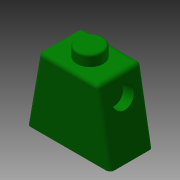
# Autodesk Inventor part: TORSO
Saved by Autodesk Inventor 2015 (Build 190159000, 159)
## iProperties
Created: 2012-05-01
Part Number: TORSO
Material: 250
Document SubType Name: Modeling
Mass: 8.54388 g
Surface Area: 9.94127 cm^2
Volume: 1.08839 cm^3
Density: 7.85 g/cm^3
Appearance: Steel
Autodesk Inventor part; units mm, degrees
ref_plane "YZ Plane" through (0, 0, 0) normal (1, 0, 0) x (0, 1, 0)
ref_plane "XZ Plane" through (0, 0, 0) normal (0, 1, 0) x (-1, 0, 0)
ref_plane "XY Plane" through (0, 0, 0) normal (0, 0, 1) x (1, 0, 0)
sketch "Sketch1" plane through (0, 0, 0) normal (0, 0, 1) x (1, 0, 0)
  line L0 (-7.72, -6.385) -> (7.72, -6.385)
  line L1 (7.72, -6.385) -> (5.4683, 6.385)
  line L2 (5.4683, 6.385) -> (-5.4683, 6.385)
  line L3 (-5.4683, 6.385) -> (-7.72, -6.385)
  point P0 (0, 0)
  point P1 (0, -6.385)
  point P2 (-6.5942, 0)
  dimension "d0" = 15.44
  dimension "d1" = 80
  dimension "d2" = 12.77
  constraints: 8 end point, 2 midpoint, 1 equal length, 1 horizontal, 1 horizontal alignment, 1 parallel, 1 vertical alignment
  measures "d0" distance of L0.start L0.end
  measures "d1" angle of L1 L0
  measures "d2" distance between parallel lines of L2 L0
extrude "Extrusion1" add sketch "Sketch1" along normal mid plane 8
sketch "Sketch2" plane through (-7.72, -6.385, 4) normal (0, -1, 0) x (1, 0, 0)
  line L0 (15.44, -8) -> (15.44, 0) projected
  line L1 (3.72, -4) -> (11.72, -4) construction
  circle A0 centre (3.72, -4) radius 2.5
  circle A1 centre (11.72, -4) radius 2.5
  point P0 (7.72, -4)
  point P1 (7.72, -4)
  dimension "d5" = 5
  dimension "d6" = 8
  constraints: 3 coincident, 2 centre point, 2 end point, 1 equal radius, 1 midpoint, 1 perpendicular
  measures "d5" diameter of A0
  measures "d6" distance of L1.start L1.end
extrude "Extrusion2" cut sketch "Sketch2" against normal blind 6
sketch "Sketch3" plane through (-5.4683, 6.385, 4) normal (0, 1, 0) x (1, 0, 0)
  circle A0 centre (5.4683, 4) radius 2.44
  dimension "d9" = 4.88
  constraints: 1 centre point, 1 coincident
  measures "d9" diameter of A0
extrude "Extrusion3" add sketch "Sketch3" along normal blind 2
fillet "Fillet1" radius 0.4 1 edges at (-2.44, 8.385, 0)
fillet "Fillet2" radius 0.75 4 edges at (-6.5942, 0, 4) (-6.5942, 0, -4) (6.5942, 0, -4) (6.5942, 0, 4)
fillet "Fillet3" radius 0.75 8 edges at (-5.2452, 6.385, -3.7803) (-5.4683, 6.385, 0) (-5.2452, 6.385, 3.7803) (0, 6.385, 4) (5.2452, 6.385, 3.7803) (5.4683, 6.385, 0) (5.2452, 6.385, -3.7803) (0, 6.385, -4)
sketch "Sketch4" plane through (-7.72, -6.385, -3.25) normal (-0.9848, 0.1736, 0) x (0, 0, 1)
  line L0 (6.5, 0) -> (0, 0) projected
  circle A0 centre (3.25, 9.5) radius 2
  point P0 (3.25, 7.6286)
  dimension "d15" = 4
  dimension "d16" = 9.5
  constraints: 1 centre point, 1 vertical alignment
  measures "d15" diameter of A0
  measures "d16" distance from line of L0 A0.centre
extrude "Extrusion4" cut sketch "Sketch4" against normal blind 2
mirror "Mirror1" about plane through (0, 0, 0) normal (1, 0, 0) of "Extrusion4"
body "Solid1"
